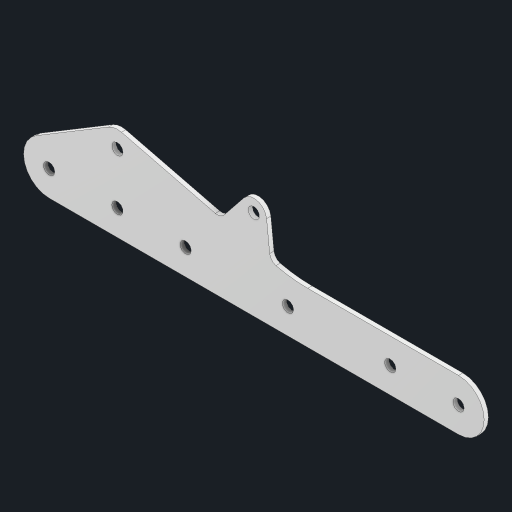
# Autodesk Inventor part: intake_gusset
Saved by Autodesk Inventor 2024 (Build 280153000, 153)
## iProperties
Created: 2023-08-21
Part Number: intake_gusset
Material: Acetal Resin, White
Document SubType Name: Modeling
Designer: Averey
Density: 1.425 g/cm^3
Appearance: Smooth - White
Author: Averey
Autodesk Inventor part; units mm, degrees
ref_plane "YZ Plane" through (0, 0, 0) normal (1, 0, 0) x (0, 1, 0)
ref_plane "XZ Plane" through (0, 0, 0) normal (0, 1, 0) x (-1, 0, 0)
ref_plane "XY Plane" through (0, 0, 0) normal (0, 0, 1) x (1, 0, 0)
sketch "Sketch1" plane through (0, 0, 0) normal (0, 0, 1) x (1, 0, 0)
  circle A0 centre (-57.8697, -2.8503) radius 2.0955
  circle A1 centre (-7.0697, -2.8503) radius 2.0955
  circle A2 centre (31.0303, -2.8503) radius 2.0955
  circle A3 centre (69.1303, -2.8503) radius 2.0955
  arc A4 (-62.7892, 5.306) -> (-57.8697, -12.3753) centre (-57.8697, -2.8503) ccw
  arc A5 (-30.9405, 22.3406) -> (-35.7494, 21.615) centre (-32.4697, 16.1775) ccw
  arc A6 (69.1303, -12.3753) -> (69.1303, 6.6747) centre (69.1303, -2.8503) ccw
  line L0 (-57.8697, -12.3753) -> (69.1303, -12.3753)
  line L1 (-62.7892, 5.306) -> (-35.1787, 21.9592)
  line L2 (69.1303, 6.6747) -> (38.4028, 6.6747)
  line L3 (-30.9405, 22.3406) -> (26.1686, 8.1699)
  arc A7 (26.1686, 8.1699) -> (38.4028, 6.6747) centre (38.4028, 57.4747) ccw
  circle A8 centre (-32.4697, 16.1775) radius 2.0955
  point P0 (0, 0)
  dimension "d0" = 4.191
  dimension "d1" = 4.191
  dimension "d2" = 4.191
  dimension "d3" = 4.191
  dimension "d4" = 50.8
  dimension "d5" = 4.191
  constraints: 9 centre point, 8 end point, 8 point on circle, 7 tangent, 3 coincident, 1 point on line, 3 other
  measures "d0" diameter of A0
  measures "d1" diameter of A1
  measures "d2" diameter of A2
  measures "d3" diameter of A3
  measures "d4" radius of A7
  measures "d5" diameter of A8
extrude "Extrusion1" add sketch "Sketch1" along normal blind 1.5875
sketch "Sketch2" plane through (-7.0697, -2.8503, 0) normal (0, 0, -1) x (-1, 0, 0)
  circle A0 centre (25.4, 0) radius 2.0955
  point P0 (-7.0697, 2.8503)
  dimension "d8" = 4.191
  constraints: 1 centre point
  measures "d8" diameter of A0
extrude "Extrusion2" cut sketch "Sketch2" against normal blind 1.5875
sketch "Sketch3" plane through (-7.0697, -2.8503, 0) normal (0, 0, -1) x (-1, 0, 0)
  line L0 (-21.6825, 26.7893) -> (-14.3342, 17.6126)
  line L1 (-30.135, 24.3239) -> (-31.2875, 13.6514)
  line L2 (-33.2384, 11.0202) -> (23.8707, 25.1909) projected
  line L3 (-33.6796, 10.9107) -> (-33.2384, 11.0202)
  arc A0 (-33.6796, 10.9107) -> (-31.2875, 13.6514) centre (-34.4442, 13.9923) ccw
  line L4 (23.8707, 25.1909) -> (-11.0912, 16.5156)
  arc A1 (-14.3342, 17.6126) -> (-11.0912, 16.5156) centre (-11.8558, 19.5972) ccw
  circle A2 centre (-25.4, 23.8125) radius 2.0955
  arc A3 (-21.6825, 26.7893) -> (-30.135, 24.3239) centre (-25.4, 23.8125) ccw
  point P0 (-7.0697, 2.8503)
  point P1 (-13.3897, 15.9453)
  point P2 (-13.0638, 16.0262)
  dimension "d19" = 3.175
  dimension "d20" = 3.175
  dimension "d21" = 4.191
  constraints: 8 end point, 6 point on circle, 6 tangent, 4 centre point, 3 point on line, 1 coincident, 1 collinear, 1 other
  measures "d19" radius of A0
  measures "d20" radius of A1
  measures "d21" diameter of A2
extrude "Extrusion3" add sketch "Sketch3" against normal blind 1.5875
sketch "Sketch5" plane through (69.1303, -2.8503, 1.5875) normal (0, 0, 1) x (1, 0, 0)
  circle A0 centre (25.4, 0) radius 2.0955
  arc A1 (25.4, -9.525) -> (25.4, 9.525) centre (25.4, 0) ccw
  line L0 (25.4, 9.525) -> (0, 9.525)
  arc A2 (0, -9.525) -> (0, 9.525) centre (0, 0) ccw projected
  line L1 (0, -9.525) -> (25.4, -9.525)
  point P0 (-69.1303, 2.8503)
  dimension "d26" = 4.191
  constraints: 4 end point, 2 centre point, 2 horizontal, 2 point on circle, 2 tangent, 1 coincident
  measures "d26" diameter of A0
extrude "Extrusion5" add sketch "Sketch5" against normal blind 1.5875
body "Solid1"
